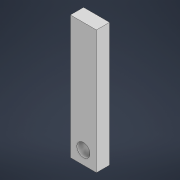
# Autodesk Inventor part: Elbow_Cube_Holder_TestFit_V2
Saved by Autodesk Inventor 2022 (Build 260153000, 153)
## iProperties
Created: 2023-05-10
Part Number: Elbow_Cube_Holder_TestFit_V2
Material: Generic
Document SubType Name: Modeling
Designer: Karl Spiteri
Density: 1 g/cm^3
Appearance: Default
Author: Karl Spiteri
Autodesk Inventor part; units mm, degrees
ref_plane "YZ Plane" through (0, 0, 0) normal (1, 0, 0) x (0, 1, 0)
ref_plane "XZ Plane" through (0, 0, 0) normal (0, 1, 0) x (-1, 0, 0)
ref_plane "XY Plane" through (0, 0, 0) normal (0, 0, 1) x (1, 0, 0)
sketch "Sketch2" plane through (0, 0, 0) normal (0, 0, 1) x (1, 0, 0)
  line L0 (0, 0) -> (-9.9, 0)
  line L1 (-9.9, 0) -> (-9.9, 105)
  line L2 (-9.9, 105) -> (0, 105)
  line L3 (0, 105) -> (0, 0)
  line L4 (-4.95, 0) -> (-4.95, 2.5)
  line L5 (-4.95, 0) -> (-2.45, 0) construction
  circle A0 centre (-4.95, 5) radius 2.5
  line L6 (-4.95, 7.5) -> (32.05, 7.5) construction
  line L7 (0, 44.5) -> (0, 0)
  line L8 (0, 0) -> (-9.9, 0)
  line L9 (-9.9, 0) -> (-9.9, 44.5)
  line L10 (0, 45.5) -> (0, 0)
  line L11 (0, 0) -> (-9.9, 0)
  line L12 (-9.9, 0) -> (-9.9, 45.5)
  line L13 (-4.95, 7.5) -> (66.05, 7.5) construction
  line L14 (-9.9, 78.5) -> (0, 78.5)
  line L15 (0, 0) -> (-9.9, 0)
  line L16 (-9.9, 0) -> (-9.9, 47)
  line L17 (-9.9, 47) -> (0, 47)
  line L18 (0, 47) -> (0, 0)
  dimension "d35" = 5
  dimension "d4" = 9.9
  dimension "d5" = 105
  dimension "d33" = 2.5
  dimension "d34" = 90
  dimension "d46" = 9.9
  dimension "d47" = 47
  constraints: 38 end point, 6 parallel, 5 horizontal, 5 point on line, 4 perpendicular, 1 midpoint, 1 vertical, 1 vertical alignment, 2 other
  measures "d4" distance of L1.end L2.end
  measures "d5" distance of L0.end L1.end
  measures "d33" distance of L4.start L4.end
  measures "d34" angle of L5 L4
  measures "d46" distance of L16.end L17.end
  measures "d47" distance of L15.end L16.end
extrude "Extrusion6" add sketch "Sketch2" along normal blind 5 contours L0 L1 L17 L3
body "Solid5"
